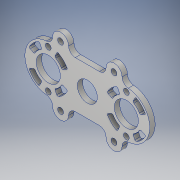
# Autodesk Inventor part: Motor Bracket
Saved by Autodesk Inventor 2019.4 (Build 234330000, 330)
## iProperties
Created: 2020-01-18
Part Number: Motor Bracket
Material: Aluminum 6061
Document SubType Name: Modeling
Designer: admin
Density: 2.7 g/cm^3
Appearance: Aluminum - Flat
Mass: 25.7313 g
Surface Area: 77.5831 cm^2
Volume: 9.53011 cm^3
Author: admin
Autodesk Inventor part; units mm, degrees
ref_plane "YZ Plane" through (0, 0, 0) normal (1, 0, 0) x (0, 1, 0)
ref_plane "XZ Plane" through (0, 0, 0) normal (0, 1, 0) x (-1, 0, 0)
ref_plane "XY Plane" through (0, 0, 0) normal (0, 0, 1) x (1, 0, 0)
sketch "Sketch1" plane through (0, 0, 0) normal (0, 0, 1) x (1, 0, 0)
  circle A0 centre (42.5576, -4.1441) radius 9
  circle A1 centre (-15.8624, -4.1441) radius 9
  line L0 (-15.8624, -4.1441) -> (42.5576, -4.1441) construction
  circle A2 centre (13.3476, -4.1441) radius 7.5
  arc A3 (42.5576, 13.3559) -> (42.5576, -21.6441) centre (42.5576, -4.1441) ccw construction
  arc A4 (-15.8624, -21.6441) -> (-15.8624, 13.3559) centre (-15.8624, -4.1441) ccw construction
  line L1 (-15.8624, 13.3559) -> (42.5576, 13.3559)
  line L2 (-15.8624, -21.6441) -> (42.5576, -21.6441)
  arc A5 (-15.8624, 13.3559) -> (-15.8624, -21.6441) centre (-15.8624, -4.1441) ccw
  arc A6 (42.5576, -21.6441) -> (42.5576, 13.3559) centre (42.5576, -4.1441) ccw
  circle A7 centre (-6.6524, 18.3559) radius 2.2
  circle A8 centre (33.3476, 18.3559) radius 2.2
  circle A9 centre (-6.6524, -26.6441) radius 2.2
  circle A10 centre (33.3476, -26.6441) radius 2.2
  circle A11 centre (-6.6524, 18.3559) radius 6
  circle A12 centre (33.3476, 18.3559) radius 6
  circle A13 centre (33.3476, -26.6441) radius 6
  circle A14 centre (-6.6524, -26.6441) radius 6
  line L3 (-6.6524, -26.6441) -> (33.3476, -26.6441) construction
  line L4 (33.3476, -26.6441) -> (33.3476, 18.3559) construction
  line L5 (33.3476, 18.3559) -> (-6.6524, 18.3559) construction
  line L6 (-6.6524, 18.3559) -> (-6.6524, -26.6441) construction
  line L7 (-6.6524, -26.6441) -> (33.3476, 18.3559) construction
  line L8 (33.3476, -26.6441) -> (-6.6524, 18.3559) construction
  circle A15 centre (42.5576, -4.1441) radius 14.5 construction
  circle A16 centre (-15.8624, -4.1441) radius 14.5 construction
  circle A17 centre (42.5576, 10.3559) radius 1.65
  circle A18 centre (42.5576, -18.6441) radius 1.65
  circle A19 centre (-15.8624, 10.3559) radius 1.65
  circle A20 centre (-15.8624, -18.6441) radius 1.65
  dimension "d1" = 18
  dimension "d2" = 18
  dimension "d3" = 15
  dimension "d4" = 58.42
  dimension "d5" = 35
  dimension "d6" = 35
  dimension "d9" = 4.4
  dimension "d10" = 4.4
  dimension "d11" = 4.4
  dimension "d12" = 4.4
  dimension "d13" = 12
  dimension "d14" = 12
  dimension "d15" = 12
  dimension "d16" = 12
  dimension "d17" = 40
  dimension "d18" = 45
  dimension "d20" = 29
  dimension "d21" = 29
  dimension "d22" = 3.3
  dimension "d23" = 3.3
  dimension "d24" = 3.3
  dimension "d25" = 3.3
  constraints: 21 centre point, 18 end point, 12 point on circle, 11 coincident, 4 tangent, 3 midpoint, 2 horizontal, 2 parallel, 1 perpendicular
  measures "d1" diameter of A0
  measures "d2" diameter of A1
  measures "d3" diameter of A2
  measures "d4" distance of L0.start L0.end
  measures "d5" diameter of A3
  measures "d6" diameter of A4
  measures "d9" diameter of A7
  measures "d10" diameter of A8
  measures "d11" diameter of A9
  measures "d12" diameter of A10
  measures "d13" diameter of A11
  measures "d14" diameter of A12
  measures "d15" diameter of A13
  measures "d16" diameter of A14
  measures "d17" distance of L4.end L5.end
  measures "d18" distance of L5.end L3.start
  measures "d20" diameter of A15
  measures "d21" diameter of A16
  measures "d22" diameter of A17
  measures "d23" diameter of A18
  measures "d24" diameter of A19
  measures "d25" diameter of A20
extrude "Extrusion1" add sketch "Sketch1" along normal blind 4
fillet "Fillet1" radius 5 8 edges at (-3.3358, 13.3559, 2) (-9.969, 13.3559, 2) (36.6642, 13.3559, 2) (30.031, 13.3559, 2) (30.031, -21.6441, 2) (36.6642, -21.6441, 2) (-3.3358, -21.6441, 2) (-9.969, -21.6441, 2)
sketch "Sketch2" plane through (0, 0, 4) normal (0, 0, 1) x (1, 0, 0)
  circle A0 centre (-15.8624, -4.1441) radius 18.65 construction
  circle A1 centre (-15.8624, -4.1441) radius 8.75 projected
  line L0 (-9.1005, -18.645) -> (-11.0868, -14.3853) projected
  arc A2 (-11.0868, -14.3853) -> (-5.6211, -8.9196) centre (-15.8624, -4.1441) ccw projected
  line L1 (-1.3615, -10.906) -> (-5.6211, -8.9196) projected
  arc A3 (-9.1005, -18.645) -> (-1.3615, -10.906) centre (-15.8624, -4.1441) ccw projected
  arc A4 (-1.3615, 2.6178) -> (-9.1005, 10.3569) centre (-15.8624, -4.1441) ccw projected
  line L2 (-5.6211, 0.6315) -> (-1.3615, 2.6178) projected
  arc A5 (-5.6211, 0.6315) -> (-11.0868, 6.0972) centre (-15.8624, -4.1441) ccw projected
  line L3 (-11.0868, 6.0972) -> (-9.1005, 10.3569) projected
  line L4 (-30.3633, -10.906) -> (-26.1037, -8.9196) projected
  arc A6 (-26.1037, -8.9196) -> (-20.638, -14.3853) centre (-15.8624, -4.1441) ccw projected
  line L5 (-22.6243, -18.645) -> (-20.638, -14.3853) projected
  arc A7 (-30.3633, -10.906) -> (-22.6243, -18.645) centre (-15.8624, -4.1441) ccw projected
  arc A8 (-22.6243, 10.3569) -> (-30.3633, 2.6178) centre (-15.8624, -4.1441) ccw projected
  line L6 (-20.638, 6.0972) -> (-22.6243, 10.3569) projected
  arc A9 (-20.638, 6.0972) -> (-26.1037, 0.6315) centre (-15.8624, -4.1441) ccw projected
  line L7 (-26.1037, 0.6315) -> (-30.3633, 2.6178) projected
  circle A10 centre (-15.8624, 10.3559) radius 1.65 projected
  circle A11 centre (-15.8624, -18.6441) radius 1.65 projected
  circle A12 centre (42.5576, -4.1441) radius 18.65 construction
  circle A13 centre (42.5576, -4.1441) radius 8.75 projected
  line L8 (49.3195, -18.645) -> (47.3332, -14.3853) projected
  arc A14 (47.3332, -14.3853) -> (52.7989, -8.9196) centre (42.5576, -4.1441) ccw projected
  line L9 (57.0585, -10.906) -> (52.7989, -8.9196) projected
  arc A15 (49.3195, -18.645) -> (57.0585, -10.906) centre (42.5576, -4.1441) ccw projected
  arc A16 (57.0585, 2.6178) -> (49.3195, 10.3569) centre (42.5576, -4.1441) ccw projected
  line L10 (52.7989, 0.6315) -> (57.0585, 2.6178) projected
  arc A17 (52.7989, 0.6315) -> (47.3332, 6.0972) centre (42.5576, -4.1441) ccw projected
  line L11 (47.3332, 6.0972) -> (49.3195, 10.3569) projected
  line L12 (28.0567, -10.906) -> (32.3163, -8.9196) projected
  arc A18 (32.3163, -8.9196) -> (37.782, -14.3853) centre (42.5576, -4.1441) ccw projected
  line L13 (35.7957, -18.645) -> (37.782, -14.3853) projected
  arc A19 (28.0567, -10.906) -> (35.7957, -18.645) centre (42.5576, -4.1441) ccw projected
  arc A20 (35.7957, 10.3569) -> (28.0567, 2.6178) centre (42.5576, -4.1441) ccw projected
  line L14 (37.782, 6.0972) -> (35.7957, 10.3569) projected
  arc A21 (37.782, 6.0972) -> (32.3163, 0.6315) centre (42.5576, -4.1441) ccw projected
  line L15 (32.3163, 0.6315) -> (28.0567, 2.6178) projected
  circle A22 centre (42.5576, 10.3559) radius 1.65 projected
  circle A23 centre (42.5576, -18.6441) radius 1.65 projected
  point P0 (0, 0)
extrude "Extrusion2" cut sketch "Sketch2" against normal through all contours L0 A2 L1 A3 | L2 A5 L3 A4 | L4 A6 L5 A7 | L6 A9 L7 A8 | L8 A14 L9 A15 | L10 A17 L11 A16 | L12 A18 L13 A19 | L14 A21 L15 A20
fillet "Fillet2" radius 1 32 edges at (-20.638, 6.0972, 2) (-26.1037, 0.6315, 2) (-30.3633, 2.6178, 2) (-22.6243, 10.3569, 2) (-11.0868, 6.0972, 2) (-9.1005, 10.3569, 2) (-1.3615, 2.6178, 2) (-5.6211, 0.6315, 2) (-1.3615, -10.906, 2) (-5.6211, -8.9196, 2) (-11.0868, -14.3853, 2) (-9.1005, -18.645, 2) (-20.638, -14.3853, 2) (-22.6243, -18.645, 2) (-30.3633, -10.906, 2) (-26.1037, -8.9196, 2) (37.782, 6.0972, 2) (35.7957, 10.3569, 2) (28.0567, 2.6178, 2) (32.3163, 0.6315, 2) (32.3163, -8.9196, 2) (28.0567, -10.906, 2) (37.782, -14.3853, 2) (35.7957, -18.645, 2) (49.3195, -18.645, 2) (47.3332, -14.3853, 2) (52.7989, -8.9196, 2) (57.0585, -10.906, 2) (52.7989, 0.6315, 2) (57.0585, 2.6178, 2) (49.3195, 10.3569, 2) (47.3332, 6.0972, 2)
sketch "Sketch3" plane through (0, 0, 4) normal (0, 0, 1) x (1, 0, 0)
  circle A0 centre (-15.8624, 10.3559) radius 1.65 projected
  circle A1 centre (-15.8624, 10.3559) radius 2.15
  circle A2 centre (42.5576, 10.3559) radius 2.15
  circle A3 centre (42.5576, 10.3559) radius 1.65 projected
  circle A4 centre (42.5576, -18.6441) radius 2.15
  circle A5 centre (-15.8624, -18.6441) radius 2.15
  circle A6 centre (-15.8624, -18.6441) radius 1.65 projected
  circle A7 centre (42.5576, -18.6441) radius 1.65 projected
  point P0 (0, 0)
  dimension "d29" = 4.3
  dimension "d30" = 4.3
  dimension "d31" = 4.3
  dimension "d32" = 4.3
  constraints: 4 centre point, 3 concentric, 1 coincident
  measures "d29" diameter of A1
  measures "d30" diameter of A2
  measures "d31" diameter of A4
  measures "d32" diameter of A5
extrude "Extrusion3" cut sketch "Sketch3" against normal blind 10
equation "\"d6\" = d5"
body "Solid1"
